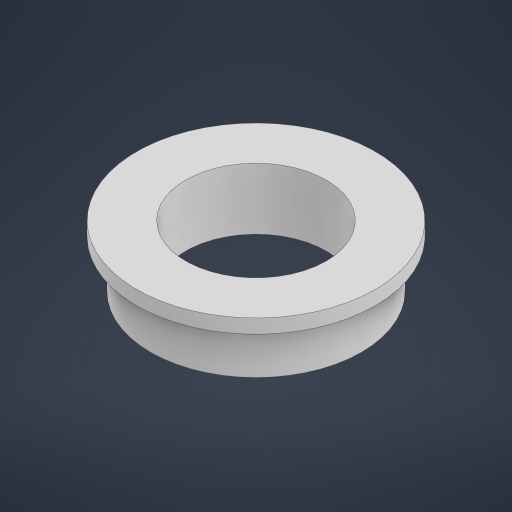
# Autodesk Inventor part: Flanged_Bearing_Izack_Waczko
Saved by Autodesk Inventor 2023 (Build 270158000, 158)
## iProperties
Created: 2023-08-25
Part Number: Flanged_Bearing_Izack_Waczko
Material: Generic
Document SubType Name: Modeling
Designer: Izack Waczko
Density: 1 g/cm^3
Appearance: Default
Author: Izack Waczko
Autodesk Inventor part; units mm, degrees
ref_plane "YZ Plane" through (0, 0, 0) normal (1, 0, 0) x (0, 1, 0)
ref_plane "XZ Plane" through (0, 0, 0) normal (0, 1, 0) x (-1, 0, 0)
ref_plane "XY Plane" through (0, 0, 0) normal (0, 0, 1) x (1, 0, 0)
sketch "Sketch1" plane through (0, 0, 0) normal (0, 0, 1) x (1, 0, 0)
  line L0 (0, 0) -> (4, 0) construction
  line L1 (4, 0) -> (4, 3.5)
  line L2 (4, 3.5) -> (6.8, 3.5)
  line L3 (4, 0) -> (6, 0)
  line L4 (6, 0) -> (6, 2.7)
  line L5 (6, 2.7) -> (6.8, 2.7)
  line L6 (6.8, 2.7) -> (6.8, 3.5)
  line L7 (0, 0) -> (0, 3.5) construction
  dimension "d0" = 4
  dimension "d1" = 3.5
  dimension "d3" = 2
  dimension "d4" = 2.7
  dimension "d5" = 0.8
  constraints: 16 end point, 3 perpendicular, 2 horizontal, 2 vertical, 1 parallel
  measures "d0" distance of L0.start L0.end
  measures "d1" distance of L0.end L1.end
  measures "d3" distance of L0.end L3.end
  measures "d4" distance of L3.end L4.end
  measures "d5" distance of L4.end L5.end
revolve "Revolution1" add sketch "Sketch1" angle 360 about axis through (0, 0, 0) along (0, 1, 0)
body "Solid1"
